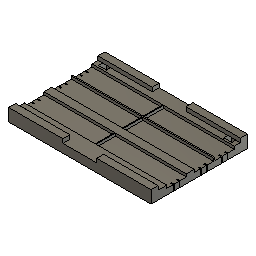
LED_panel_holder (Autodesk Fusion 360 design; units mm, degrees)
Autodesk Fusion 360 part; units mm, degrees
note: some values were not read from the file. Chosen so that the rebuilt part matches the saved one: which bodies a step acts on.
sketch "Sketch1" plane through (0, 0, 0) normal (0, 1, 0) x (1, 0, 0)
  line L0 (85, 57.5) -> (-85, 57.5)
  line L1 (-85, 57.5) -> (-85, -57.5)
  line L2 (-85, -57.5) -> (85, -57.5)
  line L3 (85, -57.5) -> (85, 57.5)
  line L4 (85, 57.5) -> (-85, -57.5) construction
  line L5 (-85, 57.5) -> (85, -57.5) construction
  circle A0 centre (-45, -27) radius 7.785 construction
  circle A1 centre (-27, -27) radius 7.785 construction
  circle A2 centre (-9, -27) radius 7.785 construction
  circle A3 centre (9, -27) radius 7.785 construction
  circle A4 centre (27, -27) radius 7.785 construction
  circle A5 centre (45, -27) radius 7.785 construction
  circle A6 centre (-45, -9) radius 7.785 construction
  circle A7 centre (-27, -9) radius 7.785 construction
  circle A8 centre (-9, -9) radius 7.785 construction
  circle A9 centre (9, -9) radius 7.785 construction
  circle A10 centre (27, -9) radius 7.785 construction
  circle A11 centre (45, -9) radius 7.785 construction
  circle A12 centre (-45, 9) radius 7.785 construction
  circle A13 centre (-27, 9) radius 7.785 construction
  circle A14 centre (-9, 9) radius 7.785 construction
  circle A15 centre (9, 9) radius 7.785 construction
  circle A16 centre (27, 9) radius 7.785 construction
  circle A17 centre (45, 9) radius 7.785 construction
  circle A18 centre (-45, 27) radius 7.785 construction
  circle A19 centre (-27, 27) radius 7.785 construction
  circle A20 centre (-9, 27) radius 7.785 construction
  circle A21 centre (9, 27) radius 7.785 construction
  circle A22 centre (27, 27) radius 7.785 construction
  circle A23 centre (45, 27) radius 7.785 construction
  line L6 (-9, 9) -> (9, -9) construction
  line L7 (9, 9) -> (-9, -9) construction
  line L8 (-9, 9) -> (9, 27) construction
  line L9 (-9, 27) -> (9, 9) construction
  line L10 (-64.3795, 18) -> (78.7409, 18) construction
  line L11 (-85, 18.75) -> (85, 18.75)
  line L12 (-85, 17.25) -> (85, 17.25)
  line L13 (-85, 42) -> (85, 42)
  line L14 (-85, -6) -> (85, -6)
  line L15 (-85, -15.375) -> (85, -15.375)
  line L16 (-85, -38.625) -> (85, -38.625)
  line L17 (27, -15.375) -> (27, -38.625) construction
  line L18 (0, 74.8277) -> (0, -83.529) construction
  line L19 (-9, -27) -> (9, -27) construction
  line L20 (-85, 18.75) -> (85, 42) construction
  line L21 (-85, -6) -> (85, 17.25) construction
  line L22 (-85, 49.15) -> (85, 49.15)
  line L23 (-85, -49.15) -> (85, -49.15)
  line L24 (-162.2656, 0) -> (88.0571, 0) construction
  line L25 (-20.15, 57.5) -> (20.15, 57.5)
  line L26 (20.15, 57.5) -> (20.15, 49.15)
  line L27 (-20.15, 49.15) -> (-20.15, 57.5)
  line L28 (-20.15, -57.5) -> (20.15, -57.5)
  line L29 (20.15, -57.5) -> (20.15, -49.15)
  line L30 (-20.15, -49.15) -> (-20.15, -57.5)
  line L31 (0.5, -57.5) -> (0.5, 42)
  line L32 (-0.5, -57.5) -> (-0.5, 42)
  point P0 (0, 18)
  point P1 (0, 30.375)
  point P2 (0, -27)
  point P3 (0, 5.625)
  dimension "d1" = 15.57
  dimension "d4" = 18
  dimension "d5" = 18
  dimension "d9" = 0.75
  dimension "d10" = 0.75
  dimension "d11" = 23.25
  dimension "d12" = 23.25
  dimension "d13" = 23.25
  dimension "d14" = 115
  dimension "d15" = 170
  dimension "d20" = 98.3
  dimension "d23" = 40.3
  dimension "d30" = 0.5
  dimension "d31" = 0.5
  constraint horizontal L0
  constraint perpendicular L0 L1
  constraint parallel L0 L2
  constraint parallel L1 L3
  constraint coincident L4 origin
  constraint coincident L5 origin
  constraint coincident A14.centre L6.start
  constraint coincident A9.centre L6.end
  constraint coincident A15.centre L7.start
  constraint coincident A8.centre L7.end
  constraint coincident origin L6
  constraint coincident origin L7
  constraint coincident A21.centre L8.end
  constraint coincident A20.centre L9.start
  constraint coincident L9 P0
  constraint coincident L8 P0
  constraint horizontal L10
  constraint coincident P0 L10
  constraint coincident L1 L11.start
  constraint horizontal L11
  constraint coincident L3 L11.end
  constraint coincident L1 L12.start
  constraint coincident L3 L12.end
  constraint horizontal L12
  constraint coincident L1 L13.start
  constraint coincident L3 L13.end
  constraint horizontal L13
  constraint coincident L1 L14.start
  constraint coincident L3 L14.end
  constraint horizontal L14
  constraint coincident L1 L15.start
  constraint coincident L3 L15.end
  constraint horizontal L15
  constraint coincident L1 L16.start
  constraint coincident L3 L16.end
  constraint horizontal L16
  constraint coincident L15 L17.start
  constraint coincident L16 L17.end
  constraint vertical L17
  constraint coincident A4.centre L17
  constraint midpoint A4.centre L17
  constraint vertical L18
  constraint coincident origin L18
  constraint coincident L18 P1
  constraint coincident A2.centre L19.start
  constraint coincident A3.centre L19.end
  constraint coincident L19 P2
  constraint coincident L18 P2
  constraint coincident P1 L20
  constraint coincident L21 P3
  constraint coincident L18 P3
  constraint coincident L1 L22.start
  constraint coincident L3 L22.end
  constraint coincident L1 L23.start
  constraint coincident L3 L23.end
  constraint horizontal L22
  constraint horizontal L23
  constraint horizontal L24
  constraint coincident origin L24
  constraint symmetric L22 L23 L24
  constraint horizontal L25
  constraint vertical L26
  constraint vertical L27
  constraint coincident L0 L25.start
  constraint horizontal L28
  constraint vertical L29
  constraint vertical L30
  constraint coincident L2 L28.start
  constraint symmetric L24 L27.start L30.start
  constraint symmetric L24 L26.end L29.end
  constraint symmetric L18 L29.end L30.start
  constraint coincident L23 L30.start
  constraint vertical L31
  constraint vertical L32
  constraint coincident L13 L31.end
  constraint coincident L28 L31.start
  constraint coincident L13 L32.end
  constraint coincident L2 L32.start
  measures "d1" diameter of A0
  measures "d9" distance of L10 L11
  measures "d10" distance of L10 L12
  measures "d11" distance of L11 L13
  measures "d12" distance of L12 L14
  measures "d13" distance of L15 L16
  measures "d14" distance of L0 L2
  measures "d15" distance of L0.start L0.end
  measures "d20" distance of L22 L23
  measures "d23" distance of L29 L30
  measures "d30" distance of L18 L31
  measures "d31" distance of L18 L32
extrude "Extrude3" add sketch "Sketch1" along normal blind 8 contours L0 L3 L22 L26 | L0 L1 L22 L27 | L2 L3 L23 L29 | L1 L2 L23 L30 makes body 1 at (-41.7667, 0, 51.9333) makes body 2 at (41.7667, 0, -51.9333) makes body 3 at (63.3833, 0, 51.9333) makes body 4 at (-63.3833, 0, -51.9333)
extrude "Extrude1" add sketch "Sketch1" along normal blind 3.25 contours L0 L22 L25 L26 L27 | L1 L3 L13 L22 | L3 L11 L12 L31 | L11 L13 L31 L32 | L11 L12 L31 L32 | L3 L14 L15 L31 | L12 L14 L31 L32 | L1 L11 L12 L32 | L14 L15 L31 L32 | L3 L16 L23 L31 | L15 L16 L31 L32 | L1 L14 L15 L32 | L16 L23 L31 L32 | L2 L23 L28 L29 L31 | L1 L16 L23 L32 | L2 L23 L28 L31 L32 | L2 L23 L28 L30 L32 bodies 1 2 4 3
extrude "Extrude2" add sketch "Sketch1" against normal blind 7 bodies 1
copy_body "Body->Comp1" bodies 1 removing the originals makes body 5 in component "panel holder"
sketch "Sketch2" plane through (0, -7, 0) normal (0, -1, 0) x (1, 0, 0)
  line L0 (-85, -57.5) -> (85, -57.5)
  line L1 (85, -57.5) -> (85, 57.5)
  line L2 (85, 57.5) -> (-85, 57.5)
  line L3 (-85, 57.5) -> (-85, -57.5)
  line L4 (70.25, -44.25) -> (79.75, -44.25)
  line L5 (79.75, -44.25) -> (79.75, -53.75)
  line L6 (79.75, -53.75) -> (70.25, -53.75)
  line L7 (70.25, -53.75) -> (70.25, -44.25)
  line L8 (70.25, 53.75) -> (79.75, 53.75)
  line L9 (79.75, 53.75) -> (79.75, 44.25)
  line L10 (79.75, 44.25) -> (70.25, 44.25)
  line L11 (70.25, 44.25) -> (70.25, 53.75)
  line L12 (-79.75, 53.75) -> (-70.25, 53.75)
  line L13 (-70.25, 53.75) -> (-70.25, 44.25)
  line L14 (-70.25, 44.25) -> (-79.75, 44.25)
  line L15 (-79.75, 44.25) -> (-79.75, 53.75)
  line L16 (-79.75, -44.25) -> (-70.25, -44.25)
  line L17 (-70.25, -44.25) -> (-70.25, -53.75)
  line L18 (-70.25, -53.75) -> (-79.75, -53.75)
  line L19 (-79.75, -53.75) -> (-79.75, -44.25)
  line L20 (0, -84.0571) -> (0, 78.4283) construction
  line L21 (119.7063, 0) -> (-101.6728, 0) construction
  line L22 (79.75, -53.75) -> (70.25, -44.25) construction
  line L23 (79.75, -44.25) -> (70.25, -53.75) construction
  line L24 (85, 38.625) -> (0.5, 38.625)
  line L25 (0.5, 15.375) -> (85, 15.375)
  line L26 (85, 38.625) -> (85, 15.375) construction
  line L27 (98.7782, 27) -> (80.2882, 27) construction
  line L28 (85, 30) -> (82, 30)
  line L29 (82, 30) -> (82, 31)
  line L30 (82, 31) -> (85, 31)
  line L31 (85, 31) -> (85, 30)
  line L32 (85, 23) -> (82, 23)
  line L33 (82, 23) -> (82, 24)
  line L34 (82, 24) -> (85, 24)
  line L35 (85, 24) -> (85, 23)
  line L36 (82, -9.625) -> (82, -8.625)
  line L37 (93.6979, -5.625) -> (75.2078, -5.625) construction
  line L38 (85, 6) -> (85, -17.25) construction
  line L39 (85, -9.625) -> (82, -9.625)
  line L40 (82, -2.625) -> (82, -1.625)
  line L41 (82, -1.625) -> (85, -1.625)
  line L42 (85, -1.625) -> (85, -2.625)
  line L43 (85, -8.625) -> (85, -9.625)
  line L44 (82, -8.625) -> (85, -8.625)
  line L45 (85, -2.625) -> (82, -2.625)
  line L46 (82, -34.375) -> (82, -33.375)
  line L47 (92.7818, -30.375) -> (75.2818, -30.375) construction
  line L48 (85, -18.75) -> (85, -42) construction
  line L49 (85, -34.375) -> (82, -34.375)
  line L50 (82, -27.375) -> (82, -26.375)
  line L51 (82, -26.375) -> (85, -26.375)
  line L52 (85, -26.375) -> (85, -27.375)
  line L53 (85, -33.375) -> (85, -34.375)
  line L54 (82, -33.375) -> (85, -33.375)
  line L55 (85, -27.375) -> (82, -27.375)
  line L56 (85, 6) -> (0.5, 6)
  line L57 (0.5, -17.25) -> (85, -17.25)
  line L58 (85, -18.75) -> (0.5, -18.75)
  line L59 (0.5, -42) -> (85, -42)
  line L60 (-82, -26.375) -> (-85, -26.375)
  line L61 (-85, 31) -> (-85, 30)
  line L62 (-82, 30) -> (-82, 31)
  line L63 (-85, -9.625) -> (-82, -9.625)
  line L64 (-85, -27.375) -> (-82, -27.375)
  line L65 (-85, -26.375) -> (-85, -27.375)
  line L66 (-85, -8.625) -> (-85, -9.625)
  line L67 (-82, -2.625) -> (-82, -1.625)
  line L68 (-85, -34.375) -> (-82, -34.375)
  line L69 (-82, 24) -> (-85, 24)
  line L70 (-85, 38.625) -> (-85, 15.375) construction
  line L71 (-82, -34.375) -> (-82, -33.375)
  line L72 (-82, -33.375) -> (-85, -33.375)
  line L73 (-85, 6) -> (-85, -17.25) construction
  line L74 (-85, 24) -> (-85, 23)
  line L75 (-82, -27.375) -> (-82, -26.375)
  line L76 (-85, -33.375) -> (-85, -34.375)
  line L77 (-82, 23) -> (-82, 24)
  line L78 (-82, -9.625) -> (-82, -8.625)
  line L79 (-85, 30) -> (-82, 30)
  line L80 (-82, -8.625) -> (-85, -8.625)
  line L81 (-82, -1.625) -> (-85, -1.625)
  line L82 (-85, 23) -> (-82, 23)
  line L83 (-85, -1.625) -> (-85, -2.625)
  line L84 (-82, 31) -> (-85, 31)
  line L85 (-85, -2.625) -> (-82, -2.625)
  point P0 (75, -49)
  point P1 (85, 38.625)
  point P2 (85, 15.375)
  point P3 (85, 27)
  point P4 (100, 1.375)
  point P5 (85, 15.375)
  point P6 (85, 38.625)
  point P7 (85, -17.25)
  point P8 (85, -5.625)
  point P9 (85, 6)
  point P10 (85, -42)
  point P11 (85, -30.375)
  point P12 (85, -18.75)
  point P13 (-85, -30.375)
  point P14 (-85, 38.625)
  point P15 (-85, 27)
  point P16 (-85, -18.75)
  point P17 (-85, 15.375)
  point P18 (-85, -18.75)
  point P19 (-85, -5.625)
  point P20 (-80.2882, 27)
  point P21 (-85, 38.625)
  point P22 (-85, 38.625)
  point P23 (-85, -17.25)
  point P24 (-85, 15.375)
  point P25 (-85, 6)
  point P26 (-85, -18.75)
  point P27 (-85, -17.25)
  point P28 (-85, 15.375)
  point P29 (-85, 6)
  dimension "d24" = 9.5
  dimension "d25" = 9.5
  dimension "d32" = 75
  dimension "d33" = 49
  dimension "d38" = 3
  dimension "d39" = 1
  dimension "d40" = 3
  dimension "d44" = 3
  dimension "d45" = 1
  dimension "d46" = 3
  dimension "d47" = 3
  dimension "d48" = 1
  dimension "d49" = 3
  constraint horizontal L4
  constraint vertical L5
  constraint horizontal L6
  constraint vertical L7
  constraint horizontal L8
  constraint vertical L9
  constraint horizontal L10
  constraint vertical L11
  constraint horizontal L12
  constraint vertical L13
  constraint horizontal L14
  constraint vertical L15
  constraint horizontal L16
  constraint vertical L17
  constraint horizontal L18
  constraint vertical L19
  constraint horizontal L21
  constraint vertical L20
  constraint symmetric L6.end L17.end L20
  constraint symmetric L4.end L16.start L20
  constraint symmetric L4.start L10.end L21
  constraint symmetric L5.end L8.end L21
  constraint symmetric L12.start L18.end L21
  constraint symmetric L13.end L16.end L21
  constraint coincident origin L20
  constraint coincident origin L21
  constraint coincident L23 P0
  constraint coincident L22 P0
  constraint coincident P6 L24
  constraint coincident L1 P6
  constraint coincident P5 L25
  constraint coincident L1 P5
  constraint coincident P6 P1
  constraint coincident P5 P2
  constraint midpoint L26 P3
  constraint coincident P3 L27
  constraint horizontal L27
  constraint horizontal L28
  constraint vertical L29
  constraint horizontal L30
  constraint vertical L31
  constraint coincident L26 L28.start
  constraint horizontal L32
  constraint vertical L33
  constraint horizontal L34
  constraint vertical L35
  constraint coincident L26 L32.start
  constraint symmetric L27 L28.end L33.end
  constraint symmetric L27 L30.end L32.start
  constraint coincident P9 L38.start
  constraint coincident P7 L38.end
  constraint midpoint P8 L38
  constraint coincident P8 L37
  constraint horizontal L37
  constraint horizontal L45
  constraint vertical L40
  constraint horizontal L41
  constraint vertical L42
  constraint coincident L42.end L38
  constraint horizontal L39
  constraint vertical L36
  constraint horizontal L44
  constraint vertical L43
  constraint coincident L39.start L38
  constraint symmetric L36.end L40.start L37
  constraint symmetric L39.start L41.end L37
  constraint coincident P12 L48.start
  constraint coincident P10 L48.end
  constraint midpoint P11 L48
  constraint coincident P11 L47
  constraint horizontal L47
  constraint horizontal L55
  constraint vertical L50
  constraint horizontal L51
  constraint vertical L52
  constraint coincident L52.end L48
  constraint horizontal L49
  constraint vertical L46
  constraint horizontal L54
  constraint vertical L53
  constraint coincident L49.start L48
  constraint symmetric L46.end L50.start L47
  constraint symmetric L49.start L51.end L47
  constraint coincident P9 L56
  constraint coincident L1 P9
  constraint coincident P7 L57
  constraint coincident P12 L58
  constraint coincident L1 P12
  constraint coincident P10 L59
  constraint symmetric L20 P6 P22
  constraint symmetric L20 P5 P28
  constraint symmetric L20 P3 P15
  constraint symmetric L20 L27.end P20
  constraint symmetric L20 L28.start L61.end
  constraint symmetric L20 L28.end L62.start
  constraint symmetric L20 L29.end L62.end
  constraint symmetric L20 L30.end L61.start
  constraint symmetric L20 L32.start L74.end
  constraint symmetric L20 L32.end L77.start
  constraint symmetric L20 L33.end L69.start
  constraint symmetric L20 L34.end L69.end
  constraint symmetric L20 P7 P27
  constraint symmetric L20 L36.start L63.end
  constraint symmetric L20 L36.end L78.end
  constraint symmetric L20 L39.start L63.start
  constraint symmetric L20 L40.start L67.start
  constraint symmetric L20 L43.start L66.start
  constraint symmetric L20 L42.end L83.end
  constraint symmetric L20 P8 P19
  constraint symmetric L20 P9 P29
  constraint symmetric L20 L41.end L81.end
  constraint symmetric L20 L40.end L67.end
  constraint symmetric L20 L46.start L68.end
  constraint symmetric L20 L46.end L71.end
  constraint symmetric L20 L49.start L68.start
  constraint symmetric L20 L50.start L64.end
  constraint symmetric L20 L53.start L72.end
  constraint symmetric L20 L52.end L64.start
  constraint symmetric L20 P11 P13
  constraint symmetric L20 P12 P26
  constraint symmetric L20 L51.end L60.end
  constraint symmetric L20 L50.end L60.start
  measures "d24" distance of L5.end L6.end
  measures "d25" distance of L4.end L5.end
  measures "d32" distance of L20 P0
  measures "d33" distance of L21 P0
  measures "d38" distance of L27 L34
  measures "d39" distance of L28 L30
  measures "d40" distance of L29.end L30.end
  measures "d44" distance of L37 L44
  measures "d45" distance of L41 L45
  measures "d46" distance of L41.end L40.end
  measures "d47" distance of L47 L54
  measures "d48" distance of L51 L55
  measures "d49" distance of L51.end L50.end
extrude "Extrude1'" cut sketch "Sketch2" along normal through all and the other way up to surface (10.25 mm away) contours L4 L5 L6 L7 | L8 L9 L10 L11 | L12 L13 L14 L15 | L16 L17 L18 L19 bodies 5 in component "panel holder"
extrude "Extrude2'" cut sketch "Sketch2" against normal through all contours L3 L68 L71 L72 L76 | L1 L46 L49 L53 L54 | L3 L60 L64 L65 L75 | L1 L50 L51 L52 L55 | L3 L63 L66 L78 L80 | L3 L67 L81 L83 L85 | L1 L36 L39 L43 L44 | L3 L69 L74 L77 L82 | L1 L40 L41 L42 L45 | L3 L61 L62 L79 L84 | L1 L32 L33 L34 L35 | L1 L28 L29 L30 L31 bodies 5 in component "panel holder"
component "panel holder" placed x (1, 0, 0) y (0, 1, 0) z (0, 0, 1) at (0, 0, 0)
equation "d11 = 22.75 mm + 0.5 mm"
equation "d12 = 22.75 mm + 0.5 mm"
equation "d13 = 22.75 mm + 0.5 mm"
equation "d16 = 2.75 mm + 0.5 mm"
equation "d20 = 98 mm + 0.3 mm"
equation "d23 = 40 mm + 0.3 mm"
